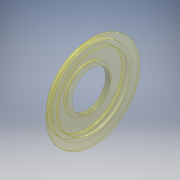
# Autodesk Inventor part: roue codeuse
Saved by Autodesk Inventor 2018.1 (Build 221171000, 171)
## iProperties
Created: 2022-06-29
Part Number: roue codeuse
Material: Generic
Document SubType Name: Modeling
Designer: Bureau
Density: 1 g/cm^3
Appearance: Default
Author: Bureau
Autodesk Inventor part; units mm, degrees
ref_plane "YZ Plane" through (0, 0, 0) normal (1, 0, 0) x (0, 1, 0)
ref_plane "XZ Plane" through (0, 0, 0) normal (0, 1, 0) x (-1, 0, 0)
ref_plane "XY Plane" through (0, 0, 0) normal (0, 0, 1) x (1, 0, 0)
sketch "Sketch1" plane through (0, 0, 0) normal (0, 0, 1) x (1, 0, 0)
  line L0 (0, 0) -> (3, 0)
  line L1 (0, 0) -> (0, 15)
  line L2 (0, 15) -> (4, 15)
  line L3 (4, 15) -> (4, 17.5)
  line L4 (4, 17.5) -> (4, 17.5)
  line L5 (4, 17.5) -> (4, 27.5)
  line L6 (4, 27.5) -> (6, 27.5)
  line L7 (6, 27.5) -> (6, 31)
  line L8 (6, 31) -> (6, 36)
  line L9 (6, 36) -> (4.5, 36)
  line L10 (4.5, 36) -> (4.5, 31)
  line L11 (4.5, 31) -> (0, 31)
  line L12 (0, 31) -> (0, 27.5)
  line L13 (0, 27.5) -> (2, 27.5)
  line L14 (2, 27.5) -> (2, 17.5)
  line L15 (2, 17.5) -> (0, 17.5)
  line L16 (0, 17.5) -> (0, 15)
  dimension "d0" = 3
  dimension "d1" = 15
  dimension "d2" = 4
  dimension "d3" = 2.5
  dimension "d4" = 0
  dimension "d5" = 10
  dimension "d6" = 2
  dimension "d7" = 3.5
  dimension "d8" = 5
  dimension "d9" = 1.5
  dimension "d10" = 31
  constraints: 34 end point, 11 perpendicular, 6 point on line, 2 horizontal, 1 vertical
  measures "d0" distance of L0.start L0.end
  measures "d1" distance of L0.start L1.end
  measures "d2" distance of L1.end L2.end
  measures "d3" distance of L2.end L3.end
  measures "d4" distance of L3.end L4.end
  measures "d5" distance of L4.end L5.end
  measures "d6" distance of L5.end L6.end
  measures "d7" distance of L6.end L7.end
  measures "d8" distance of L7.end L8.end
  measures "d9" distance of L8.end L9.end
  measures "d10" distance of L0.start L11.end
revolve "Revolution1" add sketch "Sketch1" angle 360 about axis through (0, 0, 0) along (1, 0, 0)
thread "Thread1" size "M30x1" class "6H" standard "ANSI Metric M Profile" full length
body "Solid1"
